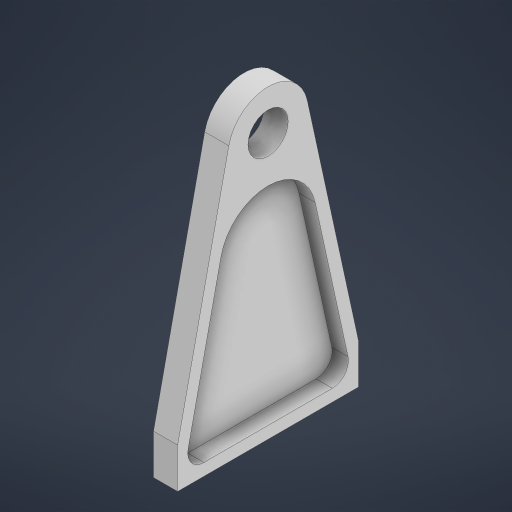
# Autodesk Inventor part: Bearing High
Saved by Autodesk Inventor 2023.2 (Build 272271000, 271)
## iProperties
Created: 2023-01-17
Part Number: Bearing High
Material: Generic
Document SubType Name: Modeling
Designer: iusti
Density: 1 g/cm^3
Appearance: Default
Author: iusti
Autodesk Inventor part; units mm, degrees
ref_plane "YZ Plane" through (0, 0, 0) normal (1, 0, 0) x (0, 1, 0)
ref_plane "XZ Plane" through (0, 0, 0) normal (0, 1, 0) x (-1, 0, 0)
ref_plane "XY Plane" through (0, 0, 0) normal (0, 0, 1) x (1, 0, 0)
sketch "Sketch1" plane through (0, 0, 0) normal (1, 0, 0) x (0, 1, 0)
  line L0 (0, 22.5) -> (0, -22.5)
  arc A0 (68.1391, -9.7685) -> (68.1391, 9.7685) centre (66, 0) ccw
  line L1 (0, 22.5) -> (10, 22.5)
  line L2 (0, -22.5) -> (10, -22.5)
  line L3 (10, -22.5) -> (68.1391, -9.7685)
  line L4 (10, 22.5) -> (68.1391, 9.7685)
  point P0 (0, 0)
  dimension "d1" = 10
  dimension "d2" = 10
  dimension "d3" = 66
  dimension "d4" = 45
  constraints: 10 end point, 2 horizontal, 2 midpoint, 2 point on circle, 2 tangent, 1 centre point, 1 horizontal alignment, 1 parallel, 1 vertical
  measures "d1" radius of A0
  measures "d2" distance of L0.start L1.end
  measures "d3" distance from line of L0 A0.centre
  measures "d4" distance between parallel lines of L2 L1
extrude "Extrusion1" add sketch "Sketch1" along normal blind 6
sketch "Sketch2" plane through (6, 0, 0) normal (1, 0, 0) x (0, 0, -1)
  line L0 (-22.5, 0) -> (22.5, 0) projected
  line L1 (22.5, 10) -> (9.7685, 68.1391) projected
  line L2 (-9.7685, 68.1391) -> (-22.5, 10) projected
  line L3 (-11.7222, 45.1931) -> (-19.8985, 7.8557)
  line L4 (-15.9911, 3) -> (15.9911, 3)
  line L5 (19.8985, 7.8557) -> (11.7222, 45.1931)
  arc A0 (11.7222, 45.1931) -> (-11.7222, 45.1931) centre (0, 42.6261) ccw
  arc A1 (-19.8985, 7.8557) -> (-15.9911, 3) centre (-15.9911, 7) ccw
  arc A2 (15.9911, 3) -> (19.8985, 7.8557) centre (15.9911, 7) ccw
  point P0 (0, 0)
  dimension "d8" = 4
  dimension "d9" = 12
  dimension "d10" = 3
  dimension "d11" = 3
  dimension "d12" = 3
  constraints: 6 end point, 6 point on circle, 6 tangent, 3 centre point, 2 parallel, 1 equal radius, 1 horizontal
  measures "d8" radius of A1
  measures "d9" radius of A0
  measures "d10" distance between parallel lines of L5 L1
  measures "d11" distance between parallel lines of L2 L3
  measures "d12" distance between parallel lines of L4 L0
extrude "Extrusion2" cut sketch "Sketch2" against normal blind 4
sketch "Sketch3" plane through (6, 0, 0) normal (1, 0, 0) x (0, 0, -1)
  arc A0 (9.7685, 68.1391) -> (-9.7685, 68.1391) centre (0, 66) ccw projected
  point P0 (0, 0)
  constraints: 1 coincident
hole "Hole1" at (6, 66, 0) direction (-1, 0, 0) diameter 10 end through all
body "Solid1"
